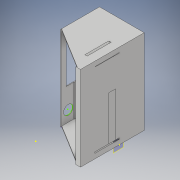
# Autodesk Inventor part: caixa interruptors
Saved by Autodesk Inventor 2019 (Build 230136000, 136)
## iProperties
Created: 2018-08-12
Part Number: caixa interruptors
Material: Genérico
Document SubType Name: Modeling
Designer: Albert Garangou Culebras
Density: 1 g/cm^3
Appearance: Valor por defecto
Author: Albert Garangou Culebras
Autodesk Inventor part; units mm, degrees
ref_plane "YZ Plane" through (0, 0, 0) normal (1, 0, 0) x (0, 1, 0)
ref_plane "XZ Plane" through (0, 0, 0) normal (0, 1, 0) x (-1, 0, 0)
ref_plane "XY Plane" through (0, 0, 0) normal (0, 0, 1) x (1, 0, 0)
sketch "Boceto15" plane through (0, 0, 0) normal (0, 1, 0) x (-1, 0, 0)
  line L0 (0, 0) -> (0, -82.5)
  line L1 (0, -82.5) -> (95.1, -82.5)
  line L2 (0, 0) -> (10, 0)
  line L3 (8.9499, -1.7021) -> (94.0499, -54.2021)
  line L4 (8.9499, -1.7021) -> (8.7796, -1.5971)
  line L5 (8.7796, -1.5971) -> (9.7649, 0)
  line L6 (10, 0) -> (9.7649, 0)
  line L7 (94.0499, -54.2021) -> (94.2201, -54.3072)
  line L8 (94.2201, -54.3072) -> (95.1, -52.8809)
  line L9 (95.1, -52.8809) -> (95.1, -82.5)
  dimension "d61" = 2
  dimension "d62" = 0.2
  constraints: 20 end point, 3 perpendicular, 2 vertical, 1 collinear, 1 horizontal, 1 point on line
  measures "d61" distance of L2.end L3.start
  measures "d62" distance of L3.end L7.end
extrude "Extrusión15" add sketch "Boceto15" along normal blind 180
sketch "Boceto16" plane through (0, 0, 0) normal (0, -1, 0) x (1, 0, 0)
  line L0 (-95.1, -52.8809) -> (-94.2201, -54.3072) projected
  line L1 (-94.2201, -54.3072) -> (-94.2201, -79.5002)
  line L2 (0, -82.5) -> (-95.1, -82.5) projected
  line L3 (-94.2201, -79.5002) -> (-2.0001, -79.5002)
  line L4 (0, 0) -> (0, -82.5) projected
  line L5 (-2.0001, -79.5002) -> (-2.0001, -1.7331)
  line L6 (-2.0001, -1.7331) -> (-9, -1.7331)
  line L7 (-94.2201, -54.3072) -> (-8.7796, -1.5971) projected
  line L8 (-94.2201, -54.3072) -> (-8.7796, -1.5971)
  dimension "d65" = 25.193
  dimension "d66" = 92.22
  constraints: 10 end point, 2 perpendicular, 2 point on line, 1 collinear, 1 horizontal, 1 parallel
  measures "d65" distance of L0.end L1.end
  measures "d66" distance of L1.end L3.end
extrude "Extrusión16" cut sketch "Boceto16" against normal blind 178
sketch "Boceto17" plane through (0, 0, 0) normal (0, -1, 0) x (1, 0, 0)
  line L0 (-9, -1.7331) -> (-2.0001, -1.7331) projected
  line L1 (-94.2201, -54.3072) -> (-9, -1.7331) projected
  line L2 (-9, -1.7331) -> (-94.2201, -54.3072)
  line L3 (-2.0001, -79.5002) -> (-94.2201, -79.5002) projected
  line L4 (-94.2201, -54.3072) -> (-94.2201, -79.5002)
  line L5 (-94.2201, -79.5002) -> (-2.0001, -79.5002)
  line L6 (-2.0001, -1.7331) -> (-2.0001, -79.5002) projected
  line L7 (-2.0001, -79.5002) -> (-2.0001, -1.7331)
  line L8 (-2.0001, -1.7331) -> (-9, -1.7331)
  point P0 (0, 0)
  constraints: 10 end point, 3 perpendicular, 2 collinear
extrude "Extrusión17" add sketch "Boceto17" against normal blind 2
sketch "Boceto18" plane through (-95.1, 0, -82.5) normal (-1, 0, 0) x (0, 0, 1)
  line L0 (0, 0) -> (29.6191, 0) projected
  line L1 (0, 0) -> (29.6191, 0)
  circle A0 centre (14.8095, 25) radius 10
  point P0 (82.5, 0)
  constraints: 2 end point, 1 centre point, 1 collinear
extrude "Extrusión18" cut sketch "Boceto18" against normal blind 17.5
sketch "Boceto23" plane through (0, 0, -82.5) normal (0, 0, -1) x (-1, 0, 0)
  line L0 (0, 0) -> (0, 180) projected
  line L1 (0, 180) -> (0, 160)
  line L2 (81, 160) -> (76, 160)
  line L3 (76, 160) -> (76, 155)
  line L4 (76, 155) -> (81, 155)
  line L5 (81, 155) -> (81, 160)
  line L6 (46, 160) -> (48, 160)
  line L7 (48, 160) -> (48, 155)
  line L8 (48, 155) -> (43, 155)
  line L9 (43, 155) -> (43, 160)
  line L10 (43, 160) -> (48, 160)
  line L11 (46, 127) -> (48, 127)
  line L12 (48, 127) -> (48, 122)
  line L13 (48, 122) -> (43, 122)
  line L14 (43, 127) -> (43, 122)
  line L15 (43, 127) -> (46, 127)
  line L16 (81, 125) -> (81, 127)
  line L17 (81, 127) -> (76, 127)
  line L18 (76, 124) -> (76, 127)
  line L19 (81, 122) -> (81, 125)
  line L20 (81, 155) -> (81, 127)
  line L21 (76, 160) -> (48, 160)
  line L22 (76, 124) -> (76, 122)
  line L23 (76, 122) -> (81, 122)
  line L24 (48, 122) -> (76, 122)
  line L25 (43, 127) -> (43, 155)
  dimension "d119" = 20
  constraints: 50 end point, 5 perpendicular, 5 vertical, 3 collinear, 3 horizontal, 2 parallel
  measures "d119" distance of L1.end L0.end
sketch "Boceto24" plane through (0, 0, -82.5) normal (0, 0, -1) x (-1, 0, 0)
  circle A0 centre (78.3646, 157.5) radius 1.5
  circle A1 centre (78.3646, 124.5) radius 1.5
  circle A2 centre (45.3646, 124.5) radius 1.5
  circle A3 centre (45.3646, 157.5) radius 1.5
  line L0 (43.3646, 157.5) -> (45.3646, 157.5)
  line L1 (43.3646, 122.5) -> (43.3646, 124.5)
  line L2 (78.3646, 122.5) -> (78.3646, 124.5)
  line L3 (43.3646, 124.5) -> (45.3646, 124.5)
  point P0 (0, 0)
  dimension "d129" = 3
  dimension "d181" = 2
  dimension "d182" = 2
  dimension "d183" = 2
  dimension "d184" = 2
  constraints: 8 end point, 4 centre point, 2 horizontal, 2 vertical
  measures "d129" diameter of A3
  measures "d181" distance of L0.start L0.end
  measures "d182" distance of L1.start L1.end
  measures "d183" distance of L2.start L2.end
  measures "d184" distance of L1.end L3.end
extrude "Extrusión24" cut sketch "Boceto24" against normal blind 10
sketch "Boceto25" plane through (0, 0, -82.5) normal (0, 0, -1) x (-1, 0, 0)
  line L0 (0, 0) -> (0, 180) projected
  line L1 (95.1, 0) -> (95.1, 180) projected
  line L2 (0, 0) -> (95.1, 0) projected
  line L3 (21.275, 42.5) -> (21.275, 12.5)
  line L4 (21.275, 42.5) -> (21.275, 72.5)
  line L5 (26.275, 72.5) -> (26.275, 12.5)
  line L6 (26.275, 12.5) -> (21.275, 12.5)
  line L7 (45.05, 72.5) -> (45.05, 12.5)
  line L8 (45.05, 12.5) -> (50.05, 12.5)
  line L9 (50.05, 12.5) -> (50.05, 72.5)
  line L10 (68.825, 72.5) -> (68.825, 12.5)
  line L11 (68.825, 12.5) -> (73.825, 12.5)
  line L12 (73.825, 12.5) -> (73.825, 63)
  line L13 (73.825, 63) -> (73.825, 72.5)
  line L14 (73.825, 72.5) -> (73.825, 85)
  line L15 (68.825, 85) -> (68.825, 72.5)
  line L16 (50.05, 72.5) -> (50.05, 85)
  line L17 (45.05, 85) -> (45.05, 72.5)
  line L18 (26.275, 72.5) -> (26.275, 85)
  line L19 (21.275, 85) -> (21.275, 72.5)
  line L20 (73.825, 85) -> (73.825, 95)
  line L21 (73.825, 95) -> (68.825, 95)
  line L22 (68.825, 95) -> (68.825, 85)
  line L23 (50.05, 85) -> (50.05, 95)
  line L24 (50.05, 95) -> (45.05, 95)
  line L25 (45.05, 95) -> (45.05, 85)
  line L26 (26.275, 85) -> (26.275, 95)
  line L27 (26.275, 95) -> (21.275, 95)
  line L28 (21.275, 95) -> (21.275, 85)
  dimension "d134" = 30
  dimension "d135" = 30
  dimension "d136" = 5
  dimension "d138" = 5
  dimension "d140" = 5
  dimension "d146" = 10
  constraints: 52 end point, 8 perpendicular, 4 vertical, 1 point on line
  measures "d134" distance of L3.start L3.end
  measures "d135" distance of L3.start L4.end
  measures "d136" distance of L4.end L5.start
  measures "d138" distance of L7.end L8.end
  measures "d140" distance of L10.end L11.end
  measures "d146" distance of L14.end L20.end
sketch "Boceto26" plane through (0, 0, 0) normal (0, -1, 0) x (1, 0, 0)
  line L0 (0, -82.5) -> (-95.1, -82.5) projected
  line L1 (-57, -82.5) -> (-29, -66.3342)
  line L2 (-57, -82.5) -> (-24.6684, -82.5) construction
  point P0 (0, 0)
  dimension "d141" = 30
  constraints: 4 end point, 1 equal length, 1 horizontal, 1 point on line
  measures "d141" angle of L2 L1
sweep "Barrido1" cut profiles "Boceto25" path "Boceto26" path curves L1
sketch "Boceto27" plane through (-2.0001, 178, -79.5002) normal (-1, 0, 0) x (0, 0, 1)
  line L0 (5, -101) -> (5, -167)
  line L1 (5, -167) -> (16, -167)
  line L2 (19, -168) -> (5, -168)
  line L3 (5, -168) -> (5, -71)
  line L4 (5, -71) -> (19, -71)
  line L5 (19, -71) -> (19, -168)
  point P0 (79.5002, -178)
  constraints: 12 end point, 2 parallel, 1 horizontal, 1 perpendicular, 1 point on line
extrude "Extrusión25" add sketch "Boceto27" against normal blind 2.0002
sketch "Boceto28" plane through (0, 0, 0) normal (0, -1, 0) x (1, 0, 0)
  line L0 (-20, -82.5) -> (-20, -9)
  line L1 (-17.5, -45.75) -> (-17.5, -65.75)
  line L2 (-22.5, -65.75) -> (-22.5, -45.75)
  line L3 (-22.5, -45.75) -> (-22.5, -30.75)
  line L4 (-22.5, -30.75) -> (-17.5, -30.75)
  line L5 (-17.5, -30.75) -> (-17.5, -45.75)
  line L6 (-22.5, -65.75) -> (-22.5, -95.75)
  line L7 (-22.5, -95.75) -> (-17.5, -95.75)
  line L8 (-17.5, -95.75) -> (-17.5, -65.1643)
  line L9 (-20, -82.5) -> (-20, -95.75)
  point P0 (0, 0)
  point P1 (0, -82.5)
  dimension "d147" = 20
  dimension "d149" = 20
  dimension "d150" = 5
  dimension "d151" = 20
  dimension "d153" = 5
  dimension "d212" = 30
  constraints: 20 end point, 3 point on line, 2 perpendicular, 1 midpoint, 1 vertical
  measures "d147" distance of point (0, -82.5) L0.start
  measures "d149" distance of L1.start L1.end
  measures "d150" distance of L1.end L2.start
  measures "d151" distance of L2.start L2.end
  measures "d153" distance of L3.end L4.end
  measures "d212" distance of L2.start L6.end
sketch "Boceto29" plane through (0, 180, 0) normal (0, 1, 0) x (1, 0, 0)
  line L0 (-20, 82.5) -> (-20, 11)
  line L1 (-17.5, 46.75) -> (-17.5, 31.75)
  line L2 (-17.5, 31.75) -> (-22.5, 31.75)
  line L3 (-22.5, 31.75) -> (-22.5, 46.75)
  line L4 (-22.5, 46.75) -> (-22.5, 66.75)
  line L5 (-17.5, 66.75) -> (-17.5, 46.75)
  line L6 (-17.5, 66.75) -> (-17.5, 96.75)
  line L7 (-22.5, 96.75) -> (-22.5, 66.75)
  line L8 (-20, 82.5) -> (-20, 96.75)
  line L9 (-22.5, 96.75) -> (-22.5, 111.75)
  line L10 (-22.5, 111.75) -> (-17.5, 111.75)
  line L11 (-17.5, 111.75) -> (-17.5, 96.75)
  line L12 (-20, 96.75) -> (-20, 111.75)
  point P0 (0, 0)
  point P1 (0, 82.5)
  point P2 (-20, 46.75)
  dimension "d156" = 15
  dimension "d157" = 5
  dimension "d158" = 15
  dimension "d160" = 5
  dimension "d211" = 15
  constraints: 26 end point, 3 perpendicular, 2 midpoint, 2 point on line, 2 vertical
  measures "d156" distance of L1.start L1.end
  measures "d157" distance of L1.end L2.end
  measures "d158" distance of L2.end L3.end
  measures "d160" distance of L4.end L5.start
  measures "d211" distance of L7.start L9.end
sketch "Boceto30" plane through (0, 0, -82.5) normal (0, 0, -1) x (-1, 0, 0)
  line L0 (0, 180) -> (95.1, 180) projected
  line L1 (25, 180) -> (6, 169.0303)
  line L2 (25, 180) -> (46.9393, 180) construction
  point P0 (0, 0)
  dimension "d161" = 150
  constraints: 4 end point, 1 equal length, 1 horizontal, 1 point on line
  measures "d161" angle of L1 L2
sweep "Barrido2" cut profiles "Boceto29" path "Boceto30" path curves L1
sketch "Boceto31" plane through (0, 0, -82.5) normal (0, 0, -1) x (-1, 0, 0)
  line L0 (40, 0) -> (17, 13.2791)
  line L1 (40, 0) -> (66.5581, 0) construction
  point P0 (0, 0)
  dimension "d164" = 150
  constraints: 4 end point, 1 equal length, 1 horizontal
  measures "d164" angle of L1 L0
sweep "Barrido3" cut profiles "Boceto28" path "Boceto31"
sketch "Boceto32" plane through (-2.0001, 178, -79.5002) normal (-1, 0, 0) x (0, 0, 1)
  line L0 (9, -172) -> (54, -172)
  line L1 (54, -172) -> (54, -161)
  line L2 (54, -161) -> (9, -161)
  line L3 (9, -161) -> (9, -172)
  line L4 (9, -15) -> (51, -15)
  line L5 (51, -15) -> (51, -3)
  line L6 (51, -3) -> (9, -3)
  line L7 (9, -3) -> (9, -15)
  point P0 (79.5002, -178)
  constraints: 16 end point, 4 parallel, 2 horizontal, 2 perpendicular, 1 point on line
extrude "Extrusión26" add sketch "Boceto32" against normal blind 2
sketch "Boceto34" plane through (-94.2201, 178, -54.3072) normal (1, 0, 0) x (0, 0, -1)
  line L0 (0, -176) -> (25.193, -176) projected
  line L1 (0, -176) -> (0, 0) projected
  line L2 (25.193, -176) -> (0, -176)
  line L3 (0, -176) -> (0, 0)
  line L4 (0, 0) -> (25.193, 0)
  line L5 (25.193, 0) -> (25.193, -176)
  point P0 (-54.3072, -178)
  constraints: 8 end point, 2 parallel, 1 horizontal, 1 perpendicular
extrude "Extrusión28" add sketch "Boceto34" along normal blind 0.5
sketch "Boceto36" plane through (0, 2, 0) normal (0, 1, 0) x (1, 0, 0)
  line L0 (-94.2201, 54.3072) -> (-9, 1.7331) projected
  line L1 (-93.7201, 54.3072) -> (-94.2201, 54.3072) projected
  line L2 (-94.2201, 54.3072) -> (-93.7201, 54.3072)
  line L3 (-94.2201, 54.3072) -> (-93.6573, 53.9599)
  line L4 (-93.7201, 54.3072) -> (-93.858, 54.0837)
  point P0 (0, 0)
  constraints: 6 end point, 2 point on line, 1 collinear, 1 perpendicular
extrude "Extrusión29" add sketch "Boceto36" along normal blind 178
sketch "Boceto37" plane through (0, 0, -82.5) normal (0, 0, -1) x (-1, 0, 0)
  circle A0 centre (78.3646, 157.5) radius 1.5 projected
  point P0 (0, 0)
extrude "Extrusión30" cut sketch "Boceto23" against normal blind 178 contours L3 L4 L20 L17 L18 L22 L24 L12 L11 L15 L25 L8 L7 L21
extrude "Extrusión31" cut sketch "Boceto18" against normal blind 53.25
sketch "Boceto40" plane through (0, 0, 0) normal (0, -1, 0) x (1, 0, 0)
  line L0 (0, -82.5) -> (0, -102.5)
  line L1 (0, -102.5) -> (0, -132.5)
  line L2 (0, -132.5) -> (-95.1, -132.5)
  line L3 (-95.1, -132.5) -> (-95.1, -82.5)
  line L4 (0, -132.5) -> (-2, -132.5)
  line L5 (0, -132.5) -> (0, -135.5)
  line L6 (0, -135.5) -> (-95.1, -135.5)
  line L7 (-95.1, -135.5) -> (-95.1, -132.5)
  line L8 (-95.1, -135.5) -> (-93.1, -135.5)
  line L9 (-93.1, -135.5) -> (-93.1, -82.5)
  line L10 (0, -135.5) -> (-2, -135.5)
  line L11 (-2, -135.5) -> (-2, -82.5)
  line L12 (0, -82.5) -> (-95.1, -82.5) projected
  line L13 (-2, -82.5) -> (0, -82.5)
  line L14 (-95.1, -82.5) -> (-93.1, -82.5)
  point P0 (0, 0)
  dimension "d194" = 20
  dimension "d195" = 30
  dimension "d196" = 2
  dimension "d197" = 3
  dimension "d198" = 2
  dimension "d199" = 2
  constraints: 28 end point, 6 perpendicular, 4 point on line, 2 collinear, 1 vertical
  measures "d194" distance of L0.start L0.end
  measures "d195" distance of L0.end L1.end
  measures "d196" distance of L1.end L4.end
  measures "d197" distance of L1.end L5.end
  measures "d198" distance of L6.end L8.end
  measures "d199" distance of L5.end L10.end
extrude "Extrusión33" add sketch "Boceto40" against normal blind 180 contours L0 L1 L2 L11 L12 | L5 L6 L11 L2 | L11 L6 L9 L2 | L9 L2 L3 L12 | L9 L6 L7 L2
ref_plane "Plano de trabajo1" through (-2, 0, -82.5) normal (-1, 0, 0) x (0, 0, 1)
sketch "Boceto42" plane through (-2, 0, -82.5) normal (-1, 0, 0) x (0, 0, 1)
  line L0 (-50, 180) -> (-50, 0) projected
  line L1 (-50, 180) -> (0, 180)
  line L2 (0, 180) -> (0, 178)
  line L3 (0, 180) -> (0, 160) projected
  line L4 (0, 178) -> (-50, 178)
  line L5 (-50, 180) -> (0, 180) projected
  line L6 (-50, 178) -> (-50, 180)
  line L7 (0, 0) -> (-50, 0) projected
  line L8 (0, 0) -> (0, 2)
  line L9 (0, 120) -> (0, 0) projected
  line L10 (0, 2) -> (-50, 2)
  line L11 (-50, 0) -> (-50, 2)
  line L12 (-50, 0) -> (0, 0)
  line L13 (82.5, 0) -> (-53, 0) projected
  line L14 (0, 2) -> (0, 0)
  dimension "d202" = 2
  dimension "d203" = 2
  constraints: 18 end point, 3 perpendicular, 3 point on line, 1 collinear, 1 horizontal, 1 parallel, 1 vertical
  measures "d202" distance of L1.end L2.end
  measures "d203" distance of L7.start L8.end
extrude "Extrusión34" add sketch "Boceto42" along normal blind 91.9
sketch "Boceto43" plane through (-2.0001, 2, -79.5002) normal (0, 0, 1) x (1, 0, 0)
  line L0 (-45.9999, 120) -> (-73.9999, 120) projected
  line L1 (-73.9999, 120) -> (-45.9999, 120)
  line L2 (-45.9999, 125) -> (-45.9999, 120) projected
  line L3 (-45.9999, 120) -> (-45.9999, 125)
  line L4 (-40.9999, 125) -> (-40.9999, 153) projected
  line L5 (-45.9999, 125) -> (-40.9999, 125)
  line L6 (-40.9999, 153) -> (-40.9999, 125) projected
  line L7 (-40.9999, 125) -> (-40.9999, 153)
  line L8 (-45.9999, 153) -> (-40.9999, 153) projected
  line L9 (-40.9999, 153) -> (-45.9999, 153)
  line L10 (-45.9999, 153) -> (-45.9999, 158)
  line L11 (-73.9999, 158) -> (-45.9999, 158) projected
  line L12 (-45.9999, 158) -> (-73.9999, 158)
  line L13 (-73.9999, 153) -> (-73.9999, 158) projected
  line L14 (-73.9999, 158) -> (-73.9999, 153)
  line L15 (-78.9999, 153) -> (-73.9999, 153) projected
  line L16 (-73.9999, 153) -> (-78.9999, 153)
  line L17 (-78.9999, 153) -> (-78.9999, 125)
  line L18 (-78.9999, 125) -> (-73.9999, 125) projected
  line L19 (-78.9999, 125) -> (-73.9999, 125)
  line L20 (-73.9999, 125) -> (-73.9999, 120)
  circle A0 centre (-43.3644, 122.5) radius 1.5 projected
  circle A1 centre (-43.3644, 122.5) radius 1.5
  circle A2 centre (-43.3644, 155.5) radius 1.5 projected
  circle A3 centre (-43.3644, 155.5) radius 1.5
  circle A4 centre (-76.3644, 155.5) radius 1.5 projected
  circle A5 centre (-76.3644, 155.5) radius 1.5
  circle A6 centre (-76.3644, 122.5) radius 1.5 projected
  circle A7 centre (-76.3644, 122.5) radius 1.5
  point P0 (2.0001, -2)
  constraints: 24 end point, 9 perpendicular, 4 centre point, 4 coincident, 2 collinear, 1 horizontal
extrude "Extrusión35" cut sketch "Boceto43" against normal blind 327
sketch "Boceto44" plane through (-2.0001, 2, -79.5002) normal (0, 0, 1) x (1, 0, 0)
  line L0 (-91.72, 176) -> (-91.72, 0) projected
  line L1 (0, 0) -> (-91.72, 0)
  line L2 (-91.0999, 0) -> (-91.0999, 176) projected
  line L3 (-91.72, 0) -> (-91.0999, 176)
  line L4 (-91.0999, 176) -> (0.619, 175.6768)
  line L5 (0, 0) -> (0, 167.0303) projected
  line L6 (0.619, 175.6768) -> (0, 0)
  point P0 (2.0001, -2)
  constraints: 8 end point, 3 perpendicular
extrude "Extrusión36" cut sketch "Boceto44" against normal blind 5 contours L1 L2 L4 L6
sketch "Boceto45" plane through (0, 0, -135.5) normal (0, 0, -1) x (-1, 0, 0)
  line L0 (95.1, 0) -> (0, 0) projected
  line L1 (47.55, 0) -> (47.55, 98.4278)
  line L2 (47.55, 0) -> (95.1, 0)
  line L3 (22.5, 0) -> (17.5, 0) projected
  line L4 (22.5, 100) -> (27.5, 100)
  line L5 (27.5, 100) -> (22.5, 100)
  line L6 (22.5, 100) -> (17.5, 100)
  line L7 (17.5, 100) -> (17.5, 0)
  line L8 (17.5, 0) -> (27.5, 0)
  line L9 (27.5, 0) -> (27.5, 100)
  line L10 (71.325, 100) -> (76.325, 100)
  line L11 (76.325, 100) -> (76.325, 0)
  line L12 (71.325, 0) -> (66.325, 0)
  line L13 (66.325, 0) -> (66.325, 100)
  line L14 (66.325, 100) -> (71.325, 100)
  line L15 (52.55, 98.4278) -> (52.55, 0)
  line L16 (47.55, 0) -> (42.55, 0)
  line L17 (42.55, 0) -> (42.55, 98.4278)
  line L18 (47.55, 98.4278) -> (47.55, 100)
  line L19 (47.55, 100) -> (42.55, 100)
  line L20 (42.55, 100) -> (42.55, 98.4278)
  line L21 (47.55, 100) -> (52.55, 100)
  line L22 (52.55, 100) -> (52.55, 98.4278)
  dimension "d213" = 100
  dimension "d214" = 100
  dimension "d215" = 5
  dimension "d216" = 5
  dimension "d217" = 5
  dimension "d218" = 10
  dimension "d219" = 5
  dimension "d220" = 5
  dimension "d221" = 5
  dimension "d222" = 5
  constraints: 42 end point, 8 perpendicular, 8 point on line, 3 horizontal, 2 collinear, 2 midpoint, 1 vertical
  measures "d213" distance of L12.start L10.start
  measures "d214" distance of L3.start L4.start
  measures "d215" distance of L4.start L4.end
  measures "d216" distance of L4.end L4.start
  measures "d217" distance of L4.start L6.end
  measures "d218" distance of L7.end L8.end
  measures "d219" distance of L10.start L10.end
  measures "d220" distance of L12.start L12.end
  measures "d221" distance of L1.end L15.start
  measures "d222" distance of L1.start L16.end
sketch "Boceto46" plane through (0, 0, 0) normal (0, -1, 0) x (1, 0, 0)
  line L0 (-43, -132.5) -> (-43, -135.5) projected
  line L1 (-43, -135.5) -> (-26.0685, -125.7246)
  line L2 (-43, -135.5) -> (-23.4492, -135.5) construction
  point P0 (0, 0)
  dimension "d223" = 30
  constraints: 4 end point, 1 equal length, 1 horizontal
  measures "d223" angle of L2 L1
sweep "Barrido4" cut profiles "Boceto45" path "Boceto46" path curves L1
sketch "Boceto47" plane through (0, 0, 0) normal (0, -1, 0) x (1, 0, 0)
  line L0 (-17.5, -135.5) -> (0, -135.5) projected
  line L1 (0, -135.5) -> (-95, -135.5)
  line L2 (-95, -135.5) -> (-95.1, -118.0444)
  line L3 (-95.1, -135.5) -> (-95.1, -52.8809) projected
  line L4 (-95.1, -118.0444) -> (0, -118.0444)
  line L5 (0, -118.0444) -> (0, -135.5)
  line L6 (-2, -82.5) -> (-2, -132.5) projected
  point P0 (0, 0)
  dimension "d226" = 95
  constraints: 8 end point, 1 collinear, 1 horizontal, 1 parallel, 1 point on line
  measures "d226" distance of L0.end L1.end
extrude "Extrusión37" add sketch "Boceto47" against normal blind 2
sketch "Boceto48" plane through (-2.0001, 178, -79.5002) normal (-1, 0, 0) x (0, 0, 1)
  line L0 (-52.9998, -176) -> (-47.0509, -176) projected
  line L1 (-52.9998, -176) -> (-52.9998, -73.5002)
  line L2 (-52.9998, 0) -> (-52.9998, -176) projected
  line L3 (-52.9998, -73.5002) -> (-32.1584, -73.5002)
  line L4 (-32.1584, -73.5002) -> (-32.1584, -176)
  line L5 (-46.2245, -176) -> (-2.9998, -176) projected
  line L6 (-52.9998, -176) -> (-32.1584, -176)
  point P0 (79.5002, -178)
  constraints: 8 end point, 2 perpendicular, 2 point on line, 1 horizontal
extrude "Extrusión38" add sketch "Boceto48" against normal blind 1
sketch "Boceto49" plane through (-95.1, 0, -52.8809) normal (-1, 0, 0) x (0, 0, 1)
  line L0 (0, 0) -> (0, 180) projected
  line L1 (0, 180) -> (-10, 180)
  line L2 (-10, 180) -> (-50, 180)
  line L3 (-50, 180) -> (-50, 51)
  line L4 (-10, 180) -> (-10, 49.6112)
  line L5 (-10, 180) -> (-10, 170)
  line L6 (-10, 170) -> (-50, 170)
  line L7 (-10, 170) -> (-10, 70)
  line L8 (-10, 70) -> (-50, 70)
  point P0 (52.8809, 0)
  dimension "d231" = 10
  dimension "d232" = 40
  dimension "d233" = 10
  dimension "d234" = 100
  constraints: 16 end point, 4 point on line, 3 perpendicular, 1 vertical
  measures "d231" distance of L0.end L1.end
  measures "d232" distance of L1.end L2.end
  measures "d233" distance of L1.end L5.end
  measures "d234" distance of L5.end L7.end
extrude "Extrusión39" cut sketch "Boceto49" against normal blind 3 contours L4 L8 L3 L6
